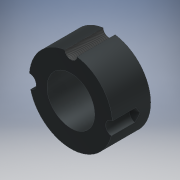
# Autodesk Inventor part: sfacciatura + tornitura piana interna ed esterna
Saved by Autodesk Inventor 2018 (Build 220112000, 112)
## iProperties
Created: 2018-08-09
Part Number: sfacciatura + tornitura piana interna ed esterna
Material: Ferro, Ghisa grigia ASTM A48 Grado 20
Document SubType Name: Modeling
Designer: carlo
Density: 7.3953 g/cm^3
Appearance: Grigio ferro
Author: carlo
Autodesk Inventor part; units mm, degrees
ref_plane "YZ Plane" through (0, 0, 0) normal (1, 0, 0) x (0, 1, 0)
ref_plane "XZ Plane" through (0, 0, 0) normal (0, 1, 0) x (-1, 0, 0)
ref_plane "XY Plane" through (0, 0, 0) normal (0, 0, 1) x (1, 0, 0)
sketch "Schizzo1" plane through (0, 0, 0) normal (0, 1, 0) x (-1, 0, 0)
  circle A0 centre (0, 0) radius 15
  circle A1 centre (0, 0) radius 40
  dimension "d0" = 30
  dimension "d1" = 80
  constraints: 2 centre point, 2 coincident
  measures "d0" diameter of A0
  measures "d1" diameter of A1
extrude "Estrusione1" add sketch "Schizzo1" against normal blind 34
sketch "Schizzo2" plane through (0, -34, 0) normal (0, -1, 0) x (1, 0, 0)
  circle A0 centre (0, 0) radius 15
  circle A1 centre (0, 0) radius 42.5
  dimension "d4" = 85
  constraints: 2 centre point, 2 coincident
  measures "d4" diameter of A1
extrude "Estrusione2" add sketch "Schizzo2" against normal blind 34
sketch "Schizzo3" plane through (0, -34, 0) normal (0, -1, 0) x (1, 0, 0)
  circle A0 centre (0, 0) radius 34.885
  line L0 (0, 41.5801) -> (0, 0)
  line L1 (0, 0) -> (-42.3383, -3.7041)
  circle A1 centre (0, 0) radius 42.5 projected
  line L2 (42.3383, -3.7041) -> (0, 0)
  point P0 (-34.7523, -3.0404)
  point P1 (34.7523, -3.0404)
  dimension "d7" = 69.77
  dimension "d8" = 95
  dimension "d9" = 95
  constraints: 6 end point, 4 point on circle, 2 point on line, 1 centre point, 1 coincident, 1 vertical
  measures "d7" diameter of A0
  measures "d8" angle of L2 L0
  measures "d9" angle of L1 L0
hole "Foro1" at (-34.7523, -34, -3.0404) at (34.7523, -34, -3.0404) direction (0, 1, 0) diameter 11.4 depth 19.8 tip angle 118 clearance for "Bullone a testa esagonale" size "7/16" standard "ANSI Unificate - Filettature"
sketch "Schizzo4" plane through (0, -34, 0) normal (0, -1, 0) x (1, 0, 0)
  circle A0 centre (0, 0) radius 34.885
  point P0 (0, 34.885)
  dimension "d17" = 69.77
  constraints: 1 coincident, 1 vertical alignment, 2 other
hole "Foro2" at (0, -34, 34.885) direction (0, 1, 0) diameter 10.262 depth 32 tip angle 118 thread size "7/16-32 UN" class "2B" standard "ANSI Unified Screw Threads"
sketch "Schizzo5" plane through (0, -34, 0) normal (0, -1, 0) x (1, 0, 0)
  circle A0 centre (0, 0) radius 20
  dimension "d25" = 40
  constraints: 1 centre point, 1 coincident
  measures "d25" diameter of A0
extrude "Estrusione3" cut sketch "Schizzo5" against normal blind 34
sketch "Schizzo6" plane through (0, 0, 0) normal (0, 1, 0) x (1, 0, 0)
  circle A0 centre (0, 0) radius 20 projected
  circle A1 centre (0, -34.885) radius 1.8024 projected
  circle A2 centre (0, 0) radius 42.5 projected
extrude "Estrusione4" cut sketch "Schizzo6" against normal blind 2
sketch "Schizzo7" plane through (0, -34, 0) normal (0, -1, 0) x (1, 0, 0)
  circle A0 centre (0, 0) radius 34.885
  circle A1 centre (0, 0) radius 42.5
  dimension "d30" = 69.77
  constraints: 2 centre point, 2 coincident
  measures "d30" diameter of A0
extrude "Estrusione5" cut sketch "Schizzo7" against normal blind 32
